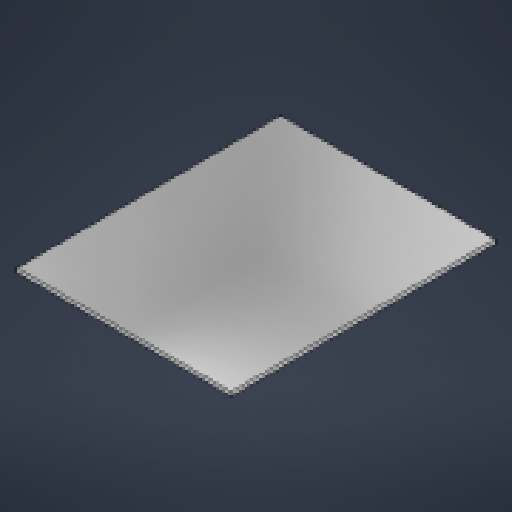
# Autodesk Inventor part: PLATE_LEFT
Saved by Autodesk Inventor 2026.1 (Build 301233020, 233B)
## iProperties
Created: 2026-03-30
Part Number: PLATE_LEFT
Material: Aluminum 6061
Document SubType Name: Sheet Metal
Designer: Owen L
Density: 2.7 g/cm^3
Sheet Metal Rule: Default
Appearance: Aluminum - Flat
Author: Owen L
Autodesk Inventor part; units mm, degrees
ref_plane "YZ Plane" through (0, 0, 0) normal (1, 0, 0) x (0, 1, 0)
ref_plane "XZ Plane" through (0, 0, 0) normal (0, 1, 0) x (-1, 0, 0)
ref_plane "XY Plane" through (0, 0, 0) normal (0, 0, 1) x (1, 0, 0)
sketch "Sketch1" plane through (0, 0, 0) normal (0, 1, 0) x (-1, 0, 0)
  line L0 (-82.55, 101.6) -> (82.55, 101.6)
  line L1 (82.55, 101.6) -> (82.55, -101.6)
  line L2 (82.55, -101.6) -> (-82.55, -101.6)
  line L3 (-82.55, -101.6) -> (-82.55, 101.6)
  line L4 (-82.55, 101.6) -> (82.55, -101.6) construction
  line L5 (82.55, 101.6) -> (-82.55, -101.6) construction
  point P0 (0, 0)
  dimension "d0" = 165.1
  dimension "d1" = 203.2
  measures "d0" distance of L1.end L2.end
  measures "d1" distance of L0.end L1.end
extrude "Plate1" add sketch "Sketch1" along normal blind 3.175
equation "\"d2\" = Thickness"
equation "\"BendRadius\" = Thickness"
equation "\"BendReliefWidth\" = Thickness"
equation "\"BendReliefDepth\" = 0.5 * Thickness"
equation "\"CornerReliefSize\" = 4 * Thickness"
equation "\"MinimumRemnant\" = 2 * Thickness"
equation "\"TransitionRadius\" = BendRadius"
equation "\"JacobiRadiusSize\" = BendRadius"
equation "\"GapSize\" = Thickness"
equation "\"Thickness\" = 3.175"
body "Solid1"
